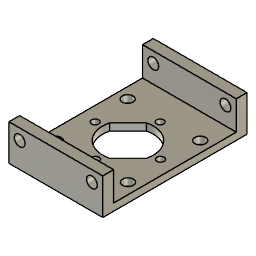
Motor Facemount (Autodesk Fusion 360 design; units mm, degrees)
Autodesk Fusion 360 part; units mm, degrees
sketch "Sketch1" plane through (0, 0, 0) normal (0, 0, 1) x (1, 0, 0)
  line L0 (0, 0) -> (26, 0)
  line L1 (26, 0) -> (26, 40)
  line L2 (26, 40) -> (0, 40)
  line L3 (0, 40) -> (0, 0)
  dimension "d1" = 26
  dimension "d2" = 40
  constraint horizontal L0
  constraint vertical L1
  constraint horizontal L2
  constraint vertical L3
  constraint coincident L0.start L3.end
  measures "d1" distance of L0.start L0.end
  measures "d2" distance of L0 L2
sketch "Sketch2" plane through (0, 0, 0) normal (0, 0, 1) x (1, 0, 0)
  circle A0 centre (23, 10) radius 1.5
  circle A1 centre (3, 10) radius 1.5
  line L0 (26, 0) -> (26, 40)
  circle A2 centre (23, 30) radius 1.5
  circle A3 centre (3.0002, 29.9091) radius 1.5
  line L1 (26, 40) -> (0, 40)
  circle A4 centre (13.0002, 28.9091) radius 1
  circle A5 centre (4.0002, 19.9091) radius 1
  circle A6 centre (13, 11) radius 1
  circle A7 centre (22, 20) radius 1
  line L2 (6.2078, 21.6931) -> (11.3069, 26.7922)
  arc A8 (6.2078, 21.6931) -> (14.6931, 13.2078) centre (13, 20) ccw
  arc A9 (19.7922, 18.3069) -> (11.3069, 26.7922) centre (13, 20) ccw
  line L3 (19.7922, 18.3069) -> (14.6931, 13.2078)
  dimension "d3" = 3
  dimension "d4" = 3
  dimension "d5" = 3
  dimension "d6" = 20
  dimension "d7" = 3
  dimension "d8" = 3
  dimension "d9" = 20
  dimension "d10" = 3
  dimension "d11" = 20
  dimension "d12" = 10
  dimension "d14" = 10
  dimension "d15" = 1
  dimension "d16" = 2
  dimension "d17" = 2
  dimension "d18" = 2
  dimension "d19" = 10
  dimension "d20" = 1
  dimension "d21" = 10
  dimension "d22" = 1
  dimension "d24" = 10
  dimension "d25" = 1
  measures "d3" diameter of A0
  measures "d4" diameter of A1
  measures "d5" distance of A0.centre L0
  measures "d6" distance of A0.centre A1.centre
  measures "d7" diameter of A2
  measures "d8" diameter of A3
  measures "d9" distance of A2.centre A3.centre
  measures "d10" distance of L0 A2.centre
  measures "d11" distance of A0.centre A2.centre
  measures "d12" distance of A2.centre L1
  measures "d14" horizontal distance of A3.centre A4.centre
  measures "d15" vertical distance of A3.centre A4.centre
  measures "d16" diameter of A5
  measures "d17" diameter of A6
  measures "d18" diameter of A7
  measures "d19" vertical distance of A3.centre A5.centre
  measures "d20" horizontal distance of A3.centre A5.centre
  measures "d21" horizontal distance of A1.centre A6.centre
  measures "d22" vertical distance of A1.centre A6.centre
  measures "d24" vertical distance of A2.centre A7.centre
  measures "d25" horizontal distance of A2.centre A7.centre
extrude "Extrude1" add sketch "Sketch1" along normal blind 2
extrude "Extrude2" cut sketch "Sketch2" along normal blind 2
sketch "Sketch3" plane through (0, 0, 2) normal (0, 0, 1) x (-1, 0, 0)
  circle A0 centre (-13.0002, -28.9091) radius 1
  circle A1 centre (-23, -10) radius 1.5
  circle A2 centre (-3, -10) radius 1.5
  circle A3 centre (-3.0002, -29.9091) radius 1.5
  circle A4 centre (-23, -30) radius 1.5
  line L0 (-6.2078, -21.6931) -> (-11.3069, -26.7922)
  arc A5 (-19.7922, -18.3069) -> (-11.3069, -26.7922) centre (-13, -20) ccw
  line L1 (-19.7922, -18.3069) -> (-14.6931, -13.2078)
  arc A6 (-6.2078, -21.6931) -> (-14.6931, -13.2078) centre (-13, -20) ccw
  circle A7 centre (-13, -11) radius 1
  circle A8 centre (-4.0002, -19.9091) radius 1
  circle A9 centre (-22, -20) radius 1
  line L2 (0, -40) -> (0, 0)
  line L3 (0, 0) -> (-26, 0)
  line L4 (-26, 0) -> (-26, -40)
  line L5 (-26, -40) -> (0, -40)
  line L6 (0, 0) -> (-26, 0)
  line L7 (-26, 0) -> (-26, -3)
  line L8 (-26, -3) -> (0, -3)
  line L9 (0, -3) -> (0, 0)
  line L10 (0, -40) -> (-26, -40)
  line L11 (-26, -40) -> (-26, -37)
  line L12 (-26, -37) -> (0, -37)
  line L13 (0, -37) -> (0, -40)
  constraint horizontal L6
  constraint vertical L7
  constraint horizontal L8
  constraint vertical L9
  constraint coincident L4 L7.end
  constraint coincident L2.end L3.start
  constraint horizontal L10
  constraint vertical L11
  constraint horizontal L12
  constraint vertical L13
  constraint coincident L4 L11.end
  constraint coincident L2.start L5.end
extrude "Extrude3" add sketch "Sketch3" along normal blind 8 contours L2 L4 L5 L10 L11 L12 L13 | L2 L3 L4 L6 L7 L8 L9
sketch "Sketch4" plane through (0, 0, 0) normal (0, -1, 0) x (1, 0, 0)
  line L0 (0, 0) -> (26, 0)
  line L1 (26, 0) -> (26, 10)
  line L2 (26, 10) -> (0, 10)
  line L3 (0, 10) -> (0, 0)
  circle A0 centre (23, 7) radius 1.5
  circle A1 centre (3, 7) radius 1.5
  dimension "d41" = 3
  dimension "d42" = 3
  dimension "d43" = 3
  dimension "d44" = 3
  dimension "d45" = 20
  measures "d41" diameter of A0
  measures "d42" diameter of A1
  measures "d43" distance of L2 A0.centre
  measures "d44" distance of L2 A1.centre
  measures "d45" distance of A0.centre A1.centre
extrude "Extrude4" cut sketch "Sketch4" against normal blind 3 contours A0 | A1
sketch "Sketch5" plane through (0, 40, 0) normal (0, 1, 0) x (-1, 0, 0)
  line L0 (-26, 0) -> (0, 0)
  line L1 (0, 0) -> (0, 10)
  line L2 (0, 10) -> (-26, 10)
  line L3 (-26, 10) -> (-26, 0)
  circle A0 centre (-3, 7) radius 1.5
  circle A1 centre (-23, 7) radius 1.5
  dimension "d48" = 3
  dimension "d49" = 3
  dimension "d50" = 20
  dimension "d51" = 3
  dimension "d52" = 3
  dimension "d53" = 3
  measures "d48" diameter of A0
  measures "d49" diameter of A1
  measures "d50" distance of A0.centre A1.centre
  measures "d51" distance of L1 A0.centre
  measures "d52" distance of L3 A1.centre
  measures "d53" distance of L2 A0.centre
extrude "Extrude5" cut sketch "Sketch5" against normal blind 3 contours A0 | A1
